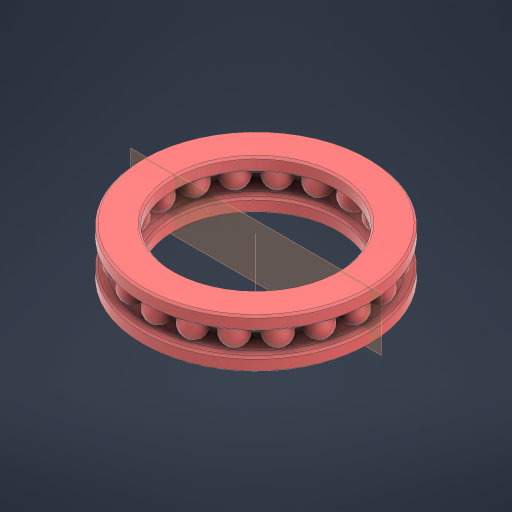
# Autodesk Inventor part: Bearing
Saved by Autodesk Inventor 2023.4 (Build 274418000, 418)
## iProperties
Created: 2025-03-29
Part Number: Bearing
Material: Generic
Document SubType Name: Modeling
Designer: Simon
Density: 1 g/cm^3
Appearance: Default
Author: Simon
Autodesk Inventor part; units mm, degrees
ref_plane "YZ Plane" through (0, 0, 0) normal (1, 0, 0) x (0, 1, 0)
ref_plane "XZ Plane" through (0, 0, 0) normal (0, 1, 0) x (-1, 0, 0)
sketch "Sketch1" plane through (0, 0, 0) normal (0, 1, 0) x (-1, 0, 0)
  circle A0 centre (0, 0) radius 21.5
  circle A1 centre (0, 0) radius 30
  dimension "d0" = 43
  dimension "d1" = 60
  constraints: 2 centre point, 2 coincident
  measures "d0" diameter of A0
  measures "d1" diameter of A1
extrude "Extrusion1" add sketch "Sketch1" along normal blind 3.62
sketch "Sketch2" plane through (0, 0, 0) normal (0, 0, 1) x (1, 0, 0)
  line L0 (-21.5, 3.62) -> (-21.5, 0) projected
  line L1 (-30, 0) -> (-30, 3.62) projected
  line L2 (-21.5, 3.62) -> (-21.5, 0) projected
  line L3 (-30, 3.62) -> (-21.5, 3.62)
  line L4 (30, 3.62) -> (-30, 3.62) projected
  line L5 (-30, 1.81) -> (-21.5, 1.81)
  line L6 (-27.95, -1.5592) -> (-23.55, -1.5592)
  line L7 (-23.55, -1.5592) -> (-23.55, 5.1792)
  line L8 (-23.55, 5.1792) -> (-27.95, 5.1792)
  line L9 (-27.95, 5.1792) -> (-27.95, -1.5592)
  line L10 (-27.95, -1.5592) -> (-23.55, 5.1792) construction
  line L11 (-23.55, -1.5592) -> (-27.95, 5.1792) construction
  line L12 (-25.75, 3.62) -> (-25.75, 3.07)
  arc A0 (-27.95, 3.62) -> (-23.55, 3.62) centre (-25.75, 7.745) ccw
  line L13 (0, 5.1792) -> (0, 7.4232)
  point P0 (0, 0)
  point P1 (-25.75, 1.81)
  dimension "d4" = 4.4
  dimension "d5" = 0.55
  constraints: 20 end point, 5 midpoint, 5 point on line, 3 point on circle, 2 parallel, 2 perpendicular, 1 centre point, 1 collinear, 1 horizontal, 1 vertical
  measures "d4" distance of L8.end L7.end
  measures "d5" distance of L12.start L12.end
revolve "Revolution1" cut sketch "Sketch2" angle 360 about axis through (0, 5.1792, 0) along (0, 1, 0) contours A0 L12 L3 | L12 A0 L3
ref_plane "Work Plane2" through (0, 6.5, 0) normal (0, -1, 0) x (1, 0, 0)
ref_plane "Work Plane1" through (0, 13, 0) normal (0, -1, 0) x (1, 0, 0)
mirror "Mirror1" about plane through (0, 6.5, 0) normal (0, -1, 0) bodies 1 separate body
sketch "Sketch3" plane through (0, 0, 0) normal (0, 0, 1) x (1, 0, 0)
  arc A0 (-25.75, 9.93) -> (-27.95, 9.38) centre (-25.75, 5.255) ccw projected
  arc A1 (-27.95, 3.62) -> (-25.75, 3.07) centre (-25.75, 7.745) ccw projected
  line L0 (-25.75, 7.745) -> (-25.75, 5.255)
  circle A2 centre (-25.75, 6.5) radius 3.25
  line L1 (-29, 6.5) -> (-22.5, 6.5)
  point P0 (0, 0)
  dimension "d8" = 6.5
  constraints: 4 end point, 2 point on circle, 1 centre point, 1 horizontal, 1 midpoint, 1 vertical
  measures "d8" diameter of A2
revolve "Revolution2" add sketch "Sketch3" angle 360 about axis through (-29, 6.5, 0) along (1, 0, 0) separate body picked at (-27.8852, 6.7593) contours L1 A2
pattern_circular "Circular Pattern1" count 20 over 360 about axis through (0, 0, 0) along (0, 1, 0) of "Revolution2" bodies 3
chamfer "Chamfer1" distance 0.5 angle 45 8 edges at (30, 0, 0) (30, 3.62, 0) (21.5, 0, 0) (21.5, 3.62, 0) (21.5, 9.38, 0) (21.5, 13, 0) (30, 13, 0) (30, 9.38, 0)
sketch "Sketch4" plane through (0, 0, 0) normal (0, 0, 1) x (1, 0, 0)
  line L0 (-30, 12.5) -> (-29.5, 13) projected
  line L1 (-22, 13) -> (-21.5, 12.5) projected
  line L2 (-21.5, 12.5) -> (-21.5, 9.88) projected
  line L3 (-21.5, 9.88) -> (-22, 9.38) projected
  line L4 (-30, 9.88) -> (-30, 12.5) projected
  line L5 (-29.5, 9.38) -> (-30, 9.88) projected
  line L6 (-30, 3.12) -> (-29.5, 3.62) projected
  line L7 (-30, 0.5) -> (-30, 3.12) projected
  line L8 (-29.5, 0) -> (-30, 0.5) projected
  line L9 (-21.5, 0.5) -> (-22, 0) projected
  line L10 (-21.5, 3.12) -> (-21.5, 0.5) projected
  line L11 (-22, 3.62) -> (-21.5, 3.12) projected
  line L12 (-29.5, 13) -> (29.5, 13) projected
  line L13 (-29.5, 13) -> (-22, 13)
  line L14 (29.5, 0) -> (-29.5, 0) projected
  line L15 (-29.5, 0) -> (-22, 0)
  line L16 (29.5, 9.38) -> (-29.5, 9.38) projected
  line L17 (-29.5, 9.38) -> (-29.5, 3.62)
  line L18 (-22, 3.62) -> (-22, 9.38)
  line L19 (-29.5, 3.62) -> (29.5, 3.62) projected
  line L20 (0, -2.6) -> (0, 15.6) projected
  line L21 (-27.95, 3.62) -> (27.95, 3.62) projected
  line L22 (-25.88, 3.62) -> (-25.88, 6.5)
  point P0 (0, 0)
  dimension "d16" = 8.5
  dimension "d17" = 3.62
  dimension "d18" = 21.5
  dimension "d19" = 5.76
  dimension "d20" = 2.88
  constraints: 10 end point, 2 collinear, 2 perpendicular, 1 parallel, 1 point on line
  measures "d16" distance between parallel lines of L10 L7
  measures "d17" distance between parallel lines of L19 L15
  measures "d18" distance between parallel lines of L10 L20
  measures "d19" distance of L5.start L6.end
  measures "d20" distance of L22.start L22.end
